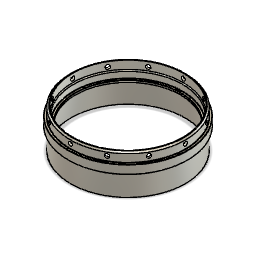
Connection-Ring-male-21.10.2024 v8 (Autodesk Fusion 360 design; units mm, degrees)
Autodesk Fusion 360 part; units mm, degrees
sketch "Skizze1" plane through (0, 0, 0) normal (0, 0, 1) x (1, 0, 0)
  line L0 (-80, 0) -> (-80, 30)
  line L1 (-80, 30) -> (-83, 30)
  line L2 (-83, 30) -> (-83, 42)
  line L3 (-83, 42) -> (-79.95, 42)
  line L4 (-79.95, 42) -> (-79.95, 53)
  line L5 (-77.95, 55) -> (-76.95, 55)
  line L6 (-76.95, 55) -> (-76.95, 42)
  line L7 (-76, 33.5) -> (-73, 33.5)
  line L8 (-73, 30.5) -> (-73, 33.5)
  line L9 (-77.95, 55) -> (-79.95, 53)
  line L10 (-80, 0) -> (-79, 0)
  line L11 (-73, 30.5) -> (-75.95, 30.5)
  line L12 (-75.95, 30.5) -> (-79, 0)
  line L13 (-76, 30) -> (-75.95, 30.5)
  line L14 (-76.95, 42) -> (-76, 42)
  line L15 (-76, 42) -> (-76, 33.5)
  dimension "d1" = 3
  dimension "d2" = 80
  dimension "d5" = 3
  dimension "d7" = 3.05
  dimension "d9" = 2
  dimension "d10" = 3
  dimension "d13" = 1
  dimension "d14" = 30
  dimension "d16" = 2
  dimension "d17" = 4
  dimension "d18" = 8.5
  dimension "d19" = 13
  dimension "d20" = 12
  dimension "d25" = 3
  constraint perpendicular L0 L1
  constraint perpendicular L1 L2
  constraint perpendicular L2 L3
  constraint perpendicular L3 L4
  constraint perpendicular L4 L5
  constraint perpendicular L3 L6
  constraint perpendicular L4 L7
  constraint perpendicular L7 L8
  constraint perpendicular L0 L10
  constraint vertical L8
  constraint perpendicular L8 L11
  constraint horizontal origin L0.start
  constraint collinear L12 L13
  constraint horizontal L0.end L13.start
  constraint perpendicular L6 L14
  constraint perpendicular L14 L15
  constraint vertical L7.start L13.start
  constraint collinear L3 L14
  measures "d1" distance of L7.end L8.start
  measures "d2" distance of origin L0
  measures "d5" distance of L4 L6
  measures "d7" distance of L2 L4
  measures "d9" distance of L4 L5.start
  measures "d10" distance of L0 L2
  measures "d13" distance of L0.start L10.end
  measures "d14" distance of L1 L10
  measures "d16" distance of L5 L4.end
  measures "d17" distance of L0.end L13.start
  measures "d18" distance of L3 L7
  measures "d19" distance of L3 L5
  measures "d20" distance of L1 L3
  measures "d25" distance of L8 L15
revolve "Drehen1" add sketch "Skizze1" angle 360 about axis through (0, 1.75, 0) along (0, 1, 0)
fillet "Abrundung1" radius 2 1 edges at (-71.7426, 42, 27.8263)
ref_plane "Arbeitsebene1" through (79.95, 47.5, 0) normal (1, 0, 0) x (0, 0, -1)
sketch "Skizze2" plane through (79.95, 0, 0) normal (1, 0, 0) x (0, 0, -1)
  line L0 (77.95, 55) -> (-77.95, 55)
  point P0 (0, 48.5)
  dimension "d27" = 6.5
  constraint vertical origin P0
  measures "d27" distance of P0 L0
hole "Bohrung1" at (79.95, 48.5, 0) direction (-1, 0, 0) diameter 5.5 depth 16 tip angle 118
pattern_circular "C-Anordnung1" count 12 over 360 about axis through (0, 1.75, 0) along (0, 1, 0) of "Bohrung1"
chamfer "Fase1" distance 0.4 angle 45 9 edges at (-77.3832, 42, 30.0141) (-77.3832, 30, 30.0141) (-73.6539, 0, 28.5676) (-70.8103, 30.5, 27.4647) (-68.0599, 30.5, 26.3979) (-70.8569, 33.5, 27.4828) (-74.5396, 42, 28.9112) (-74.5862, 0, 28.9292) (-68.0599, 33.5, 26.3979)
fillet "Abrundung2" radius 2 1 edges at (-74.5862, 30, 28.9292)
equation "d2 = ( 160 / 2 ) * 1 mm"
equation "d18 = 15 mm - d19 / 2"
